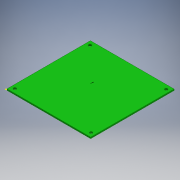
# Autodesk Inventor part: メイン基板
Saved by Autodesk Inventor 2018 (Build 220112000, 112)
## iProperties
Created: 2018-08-18
Part Number: メイン基板
Material: 一般
Document SubType Name: Modeling
Designer: shun2
Density: 1 g/cm^3
Appearance: 濃い緑
Author: shun2
Autodesk Inventor part; units mm, degrees
ref_plane "YZ Plane" through (0, 0, 0) normal (1, 0, 0) x (0, 1, 0)
ref_plane "XZ Plane" through (0, 0, 0) normal (0, 1, 0) x (-1, 0, 0)
ref_plane "XY Plane" through (0, 0, 0) normal (0, 0, 1) x (1, 0, 0)
sketch "スケッチ1" plane through (0, 0, 0) normal (0, 0, 1) x (1, 0, 0)
  line L0 (0, 100) -> (99.04, 100)
  line L1 (99.04, 100) -> (99.04, 1.27)
  line L2 (99.04, 1.27) -> (0, 1.27)
  line L3 (0, 1.27) -> (0, 100)
  circle A0 centre (94.6564, 95.0331) radius 1.6
  circle A1 centre (94.6564, 6.1331) radius 1.6
  circle A2 centre (4.4864, 6.1331) radius 1.6
  circle A3 centre (4.4864, 95.0331) radius 1.6
  point P0 (0, 0)
  dimension "d2" = 3.2
  dimension "d3" = 3.2
  dimension "d4" = 3.2
  dimension "d5" = 3.2
  constraints: 8 end point, 4 centre point, 2 parallel, 1 horizontal, 1 perpendicular
  measures "d2" diameter of A0
  measures "d3" diameter of A1
  measures "d4" diameter of A2
  measures "d5" diameter of A3
extrude "押し出し2" add sketch "スケッチ1" along normal blind 1.6
sketch "スケッチ2" plane through (0, 0, 1.6) normal (0, 0, 1) x (1, 0, 0)
  line L0 (43.0744, 59.3857) -> (45.1715, 59.3857) construction
  line L1 (45.1715, 59.3857) -> (45.1715, 55.7795) construction
  line L2 (45.1715, 55.7795) -> (43.0744, 55.7795) construction
  line L3 (43.0744, 55.7795) -> (43.0744, 59.3857) construction
  point P0 (0, 0)
  constraints: 2 other
